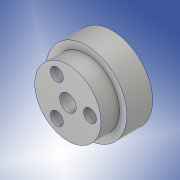
# Autodesk Inventor part: WA005
Saved by Autodesk Inventor 2017 SP1 (Build 210196100, 196)
## iProperties
Created: 2017-08-06
Part Number: WA005
Material: Aluminum 6061
Document SubType Name: Modeling
Designer: Zach
Density: 2.7 g/cm^3
Appearance: Aluminum - Flat
Author: Zach
Autodesk Inventor part; units mm, degrees
ref_plane "YZ Plane" through (0, 0, 0) normal (1, 0, 0) x (0, 1, 0)
ref_plane "XZ Plane" through (0, 0, 0) normal (0, 1, 0) x (-1, 0, 0)
ref_plane "XY Plane" through (0, 0, 0) normal (0, 0, 1) x (1, 0, 0)
sketch "Sketch1" plane through (0, 0, 0) normal (0, 0, 1) x (1, 0, 0)
  circle A0 centre (0, 0) radius 11
  dimension "d0" = 22
  constraints: 1 centre point, 1 coincident
  measures "d0" diameter of A0
extrude "Extrusion1" add sketch "Sketch1" along normal blind 7
sketch "Sketch2" plane through (0, 0, 7) normal (0, 0, 1) x (1, 0, 0)
  circle A0 centre (0, 0) radius 9
  dimension "d3" = 18
  constraints: 1 centre point, 1 coincident
  measures "d3" diameter of A0
extrude "Extrusion2" add sketch "Sketch2" along normal blind 5
sketch "Sketch3" plane through (0, 0, 12) normal (0, 0, 1) x (1, 0, 0)
  circle A0 centre (0, 0) radius 2.25
  circle A1 centre (6, 0) radius 1.75
  circle A2 centre (-3, 5.1962) radius 1.75
  circle A3 centre (-3, -5.1962) radius 1.75
  dimension "d6" = 4.5
  dimension "d7" = 3.5
  dimension "d8" = 6
  dimension "d11" = 360
  constraints: 4 centre point, 1 coincident, 1 horizontal alignment, 7 other
  measures "d6" diameter of A0
  measures "d7" diameter of A1
  measures "d8" distance of A1.centre point (0, 0)
extrude "Extrusion3" cut sketch "Sketch3" against normal through all
body "Solid1"
